Autodesk Inventor part; units mm, degrees
(part 2 of 2)
extrude "Extrusion4" cut sketch "Sketch10" against normal through all contours L3 L2 L1 L0 | L7 L6 L5 L4 | L13 L12 L11 L10 | L17 L16 L15 L14 | L69 L68 L67 L66 | L73 L72 L71 L70 | L77 L76 L75 L74 | L81 L80 L79 L78 | L85 L84 L83 L82 | L89 L88 L87 L86 | L93 L92 L91 L90 | L97 L96 L95 L94 | L101 L100 L99 L98 | L105 L104 L103 L102 | L109 L108 L107 L106 | L113 L112 L111 L110 | L117 L116 L115 L114 | L121 L120 L119 L118 | L125 L124 L123 L122 | L129 L128 L127 L126 | L133 L132 L131 L130 | L137 L136 L135 L134 | L141 L140 L139 L138 | L145 L144 L143 L142 | L197 L196 L195 L194 | L201 L200 L199 L198 | L205 L204 L203 L202 | L209 L208 L207 L206 | L213 L212 L211 L210 | L217 L216 L215 L214 | L221 L220 L219 L218 | L225 L224 L223 L222 | L229 L228 L227 L226 | L233 L232 L231 L230 | L237 L236 L235 L234 | L241 L240 L239 L238 | L245 L244 L243 L242 | L249 L248 L247 L246 | L253 L252 L251 L250 | L257 L256 L255 L254 | L261 L260 L259 L258 | L265 L264 L263 L262 | L269 L268 L267 L266 | L273 L272 L271 L270 | L325 L324 L323 L322 | L329 L328 L327 L326 | L333 L332 L331 L330 | L337 L336 L335 L334 | L341 L340 L339 L338 | L345 L344 L343 L342 | L349 L348 L347 L346 | L353 L352 L351 L350 | L357 L356 L355 L354 | L361 L360 L359 L358 | L365 L364 L363 L362 | L369 L368 L367 L366 | L373 L372 L371 L370 | L377 L376 L375 L374 | L381 L380 L379 L378 | L385 L384 L383 L382 | L389 L388 L387 L386 | L393 L392 L391 L390 | L397 L396 L395 L394 | L401 L400 L399 L398 | L453 L452 L451 L450 | L457 L456 L455 L454 | L461 L460 L459 L458 | L465 L464 L463 L462 | L469 L468 L467 L466 | L473 L472 L471 L470 | L477 L476 L475 L474 | L481 L480 L479 L478 | L485 L484 L483 L482 | L489 L488 L487 L486 | L493 L492 L491 L490 | L497 L496 L495 L494 | L501 L500 L499 L498 | L505 L504 L503 L502 | L509 L508 L507 L506 | L513 L512 L511 L510 | L517 L516 L515 L514 | L521 L520 L519 L518 | L525 L524 L523 L522 | L529 L528 L527 L526 | L533 L532 L531 L530 | L561 L560 L559 L558 | L565 L564 L563 L562 | L585 L584 L583 L582 | L589 L588 L587 L586 | L617 L616 L615 L614 | L621 L620 L619 L618 | L641 L640 L639 L638 | L645 L644 L643 L642 | L649 L648 L647 L646 | L653 L652 L651 L650 | L657 L656 L655 L654 | L661 L660 L659 L658 | L665 L664 L663 L662 | L669 L668 L667 L666 | L673 L672 L671 L670 | L677 L676 L675 L674 | L681 L680 L679 L678 | L685 L684 L683 L682 | L689 L688 L687 L686 | L693 L692 L691 L690 | L697 L696 L695 L694 | L701 L700 L699 L698 | L705 L704 L703 L702 | L709 L708 L707 L706 | L713 L712 L711 L710 | L717 L716 L715 L714 | L721 L720 L719 L718 | L725 L724 L723 L722 | L729 L728 L727 L726 | L733 L732 L731 L730 | L737 L736 L735 L734 | L741 L740 L739 L738 | L745 L744 L743 L742 | L749 L748 L747 L746 | L753 L752 L751 L750 | L757 L756 L755 L754 | L761 L760 L759 L758 | L765 L764 L763 L762 | L769 L768 L767 L766 | L773 L772 L771 L770 | L777 L776 L775 L774 | L781 L780 L779 L778 | L785 L784 L783 L782 | L789 L788 L787 L786 | L793 L792 L791 L790 | L797 L796 L795 L794 | L801 L800 L799 L798 | L805 L804 L803 L802 | L809 L808 L807 L806 | L813 L812 L811 L810 | L817 L816 L815 L814 | L821 L820 L819 L818 | L825 L824 L823 L822 | L829 L828 L827 L826 | L833 L832 L831 L830 | L837 L836 L835 L834 | L841 L840 L839 L838 | L845 L844 L843 L842 | L849 L848 L847 L846 | L853 L852 L851 L850 | L857 L856 L855 L854 | L861 L860 L859 L858 | L865 L864 L863 L862 | L869 L868 L867 L866 | L873 L872 L871 L870 | L877 L876 L875 L874 | L881 L880 L879 L878 | L885 L884 L883 L882 | L889 L888 L887 L886 | L893 L892 L891 L890 | L897 L896 L895 L894 | L901 L900 L899 L898 | L903 L904 L905 L906 | L910 L909 L908 L907 | L914 L913 L912 L911 | L918 L917 L916 L915 | L922 L921 L920 L919 | L926 L925 L924 L923 | L930 L929 L928 L927 | L934 L933 L932 L931 | L938 L937 L936 L935 | L942 L941 L940 L939 | L946 L945 L944 L943
sketch "Sketch15" plane through (0, 4, 0) normal (0, 1, 0) x (1, 0, 0)
  line L0 (-51, 1.5) -> (-22, 1.5)
  line L1 (-22, 1.5) -> (-22, 30.5)
  line L2 (-22, 30.5) -> (-51, 30.5)
  line L3 (-51, 30.5) -> (-51, 1.5)
  line L4 (-39.75, 1.5) -> (-48.25, 1.5) projected
  line L5 (-62, 131.5) -> (-62, -129.5) projected
  line L6 (-51, 31.5) -> (-22, 31.5)
  line L7 (-22, 31.5) -> (-22, 60.5)
  line L8 (-22, 60.5) -> (-51, 60.5)
  line L9 (-51, 60.5) -> (-51, 31.5)
  line L10 (-51, 61.5) -> (-22, 61.5)
  line L11 (-22, 61.5) -> (-22, 90.5)
  line L12 (-22, 90.5) -> (-51, 90.5)
  line L13 (-51, 90.5) -> (-51, 61.5)
  line L14 (-51, 91.5) -> (-22, 91.5)
  line L15 (-22, 91.5) -> (-22, 120.5)
  line L16 (-22, 120.5) -> (-51, 120.5)
  line L17 (-51, 120.5) -> (-51, 91.5)
  line L18 (-39.75, 31.5) -> (-48.25, 31.5) projected
  line L19 (-39.75, 61.5) -> (-48.25, 61.5) projected
  line L20 (-39.75, 91.5) -> (-48.25, 91.5) projected
  point P0 (0, 0)
  dimension "d162" = 29
  dimension "d163" = 0
  dimension "d164" = 11
  dimension "d165" = 29
  dimension "d166" = 29
  dimension "d167" = 29
  dimension "d168" = 29
  dimension "d169" = 0
  dimension "d170" = 0
  dimension "d171" = 0
  dimension "d172" = 11
  constraints: 32 end point, 8 parallel, 5 point on line, 4 horizontal, 4 perpendicular
  measures "d162" distance of L2.end L0.start
  measures "d163" distance between parallel lines of L4 L0
  measures "d164" distance between parallel lines of L5 L3
  measures "d165" distance of L1.end L2.end
  measures "d166" distance of L8.end L6.start
  measures "d167" distance of L12.end L10.start
  measures "d168" distance of L16.end L14.start
  measures "d169" distance between parallel lines of L18 L6
  measures "d170" distance between parallel lines of L19 L10
  measures "d171" distance between parallel lines of L20 L14
  measures "d172" distance between parallel lines of L5 L9
extrude "Extrusion5" cut sketch "Sketch15" against normal through all
sketch "Sketch16" plane through (0, 4, 0) normal (0, 1, 0) x (1, 0, 0)
  line L0 (-51, 0.5) -> (-51, -88.5) projected
  line L1 (-51, 0.5) -> (-22, 0.5)
  line L2 (-22, 0.5) -> (-22, 120.5)
  line L3 (-22, 120.5) -> (-51, 120.5)
  line L4 (-51, 120.5) -> (-51, 0.5)
  point P0 (0, 0)
  constraints: 8 end point, 2 parallel, 1 horizontal, 1 perpendicular
extrude "Extrusion6" cut sketch "Sketch16" against normal through all
sketch "Sketch18" plane through (0, 4, 0) normal (0, 1, 0) x (1, 0, 0)
  line L0 (-38.5, -115.5) -> (-37, -115.5)
  line L1 (-37, -115.5) -> (-37, -107.5)
  line L2 (-37, -107.5) -> (-38.5, -107.5)
  line L3 (-38.5, -107.5) -> (-38.5, -115.5)
  line L4 (-39.75, -118.5) -> (-48.25, -118.5) projected
  line L5 (-39.75, -117) -> (-39.75, -118.5) projected
  line L6 (-23.5, -115.5) -> (-22, -115.5)
  line L7 (-22, -115.5) -> (-22, -107.5)
  line L8 (-22, -107.5) -> (-23.5, -107.5)
  line L9 (-23.5, -107.5) -> (-23.5, -115.5)
  line L10 (-8.5, -115.5) -> (-7, -115.5)
  line L11 (-7, -115.5) -> (-7, -107.5)
  line L12 (-7, -107.5) -> (-8.5, -107.5)
  line L13 (-8.5, -107.5) -> (-8.5, -115.5)
  line L14 (6.5, -115.5) -> (8, -115.5)
  line L15 (8, -115.5) -> (8, -107.5)
  line L16 (8, -107.5) -> (6.5, -107.5)
  line L17 (6.5, -107.5) -> (6.5, -115.5)
  line L18 (21.5, -115.5) -> (23, -115.5)
  line L19 (23, -115.5) -> (23, -107.5)
  line L20 (23, -107.5) -> (21.5, -107.5)
  line L21 (21.5, -107.5) -> (21.5, -115.5)
  line L22 (36.5, -115.5) -> (38, -115.5)
  line L23 (38, -115.5) -> (38, -107.5)
  line L24 (38, -107.5) -> (36.5, -107.5)
  line L25 (36.5, -107.5) -> (36.5, -115.5)
  line L26 (51.5, -115.5) -> (53, -115.5)
  line L27 (53, -115.5) -> (53, -107.5)
  line L28 (53, -107.5) -> (51.5, -107.5)
  line L29 (51.5, -107.5) -> (51.5, -115.5)
  line L30 (-38.5, -100.5) -> (-37, -100.5)
  line L31 (-37, -100.5) -> (-37, -92.5)
  line L32 (-37, -92.5) -> (-38.5, -92.5)
  line L33 (-38.5, -92.5) -> (-38.5, -100.5)
  line L34 (-23.5, -100.5) -> (-22, -100.5)
  line L35 (-22, -100.5) -> (-22, -92.5)
  line L36 (-22, -92.5) -> (-23.5, -92.5)
  line L37 (-23.5, -92.5) -> (-23.5, -100.5)
  line L38 (-8.5, -100.5) -> (-7, -100.5)
  line L39 (-7, -100.5) -> (-7, -92.5)
  line L40 (-7, -92.5) -> (-8.5, -92.5)
  line L41 (-8.5, -92.5) -> (-8.5, -100.5)
  line L42 (6.5, -100.5) -> (8, -100.5)
  line L43 (8, -100.5) -> (8, -92.5)
  line L44 (8, -92.5) -> (6.5, -92.5)
  line L45 (6.5, -92.5) -> (6.5, -100.5)
  line L46 (21.5, -100.5) -> (23, -100.5)
  line L47 (23, -100.5) -> (23, -92.5)
  line L48 (23, -92.5) -> (21.5, -92.5)
  line L49 (21.5, -92.5) -> (21.5, -100.5)
  line L50 (36.5, -100.5) -> (38, -100.5)
  line L51 (38, -100.5) -> (38, -92.5)
  line L52 (38, -92.5) -> (36.5, -92.5)
  line L53 (36.5, -92.5) -> (36.5, -100.5)
  line L54 (51.5, -100.5) -> (53, -100.5)
  line L55 (53, -100.5) -> (53, -92.5)
  line L56 (53, -92.5) -> (51.5, -92.5)
  line L57 (51.5, -92.5) -> (51.5, -100.5)
  line L58 (-38.5, -85.5) -> (-37, -85.5)
  line L59 (-37, -85.5) -> (-37, -77.5)
  line L60 (-37, -77.5) -> (-38.5, -77.5)
  line L61 (-38.5, -77.5) -> (-38.5, -85.5)
  line L62 (-23.5, -85.5) -> (-22, -85.5)
  line L63 (-22, -85.5) -> (-22, -77.5)
  line L64 (-22, -77.5) -> (-23.5, -77.5)
  line L65 (-23.5, -77.5) -> (-23.5, -85.5)
  line L66 (-8.5, -85.5) -> (-7, -85.5)
  line L67 (-7, -85.5) -> (-7, -77.5)
  line L68 (-7, -77.5) -> (-8.5, -77.5)
  line L69 (-8.5, -77.5) -> (-8.5, -85.5)
  line L70 (6.5, -85.5) -> (8, -85.5)
  line L71 (8, -85.5) -> (8, -77.5)
  line L72 (8, -77.5) -> (6.5, -77.5)
  line L73 (6.5, -77.5) -> (6.5, -85.5)
  line L74 (21.5, -85.5) -> (23, -85.5)
  line L75 (23, -85.5) -> (23, -77.5)
  line L76 (23, -77.5) -> (21.5, -77.5)
  line L77 (21.5, -77.5) -> (21.5, -85.5)
  line L78 (36.5, -85.5) -> (38, -85.5)
  line L79 (38, -85.5) -> (38, -77.5)
  line L80 (38, -77.5) -> (36.5, -77.5)
  line L81 (36.5, -77.5) -> (36.5, -85.5)
  line L82 (51.5, -85.5) -> (53, -85.5)
  line L83 (53, -85.5) -> (53, -77.5)
  line L84 (53, -77.5) -> (51.5, -77.5)
  line L85 (51.5, -77.5) -> (51.5, -85.5)
  line L86 (-38.5, -70.5) -> (-37, -70.5)
  line L87 (-37, -70.5) -> (-37, -62.5)
  line L88 (-37, -62.5) -> (-38.5, -62.5)
  line L89 (-38.5, -62.5) -> (-38.5, -70.5)
  line L90 (-23.5, -70.5) -> (-22, -70.5)
  line L91 (-22, -70.5) -> (-22, -62.5)
  line L92 (-22, -62.5) -> (-23.5, -62.5)
  line L93 (-23.5, -62.5) -> (-23.5, -70.5)
  line L94 (-8.5, -70.5) -> (-7, -70.5)
  line L95 (-7, -70.5) -> (-7, -62.5)
  line L96 (-7, -62.5) -> (-8.5, -62.5)
  line L97 (-8.5, -62.5) -> (-8.5, -70.5)
  line L98 (6.5, -70.5) -> (8, -70.5)
  line L99 (8, -70.5) -> (8, -62.5)
  line L100 (8, -62.5) -> (6.5, -62.5)
  line L101 (6.5, -62.5) -> (6.5, -70.5)
  line L102 (21.5, -70.5) -> (23, -70.5)
  line L103 (23, -70.5) -> (23, -62.5)
  line L104 (23, -62.5) -> (21.5, -62.5)
  line L105 (21.5, -62.5) -> (21.5, -70.5)
  line L106 (36.5, -70.5) -> (38, -70.5)
  line L107 (38, -70.5) -> (38, -62.5)
  line L108 (38, -62.5) -> (36.5, -62.5)
  line L109 (36.5, -62.5) -> (36.5, -70.5)
  line L110 (51.5, -70.5) -> (53, -70.5)
  line L111 (53, -70.5) -> (53, -62.5)
  line L112 (53, -62.5) -> (51.5, -62.5)
  line L113 (51.5, -62.5) -> (51.5, -70.5)
  line L114 (-38.5, -55.5) -> (-37, -55.5)
  line L115 (-37, -55.5) -> (-37, -47.5)
  line L116 (-37, -47.5) -> (-38.5, -47.5)
  line L117 (-38.5, -47.5) -> (-38.5, -55.5)
  line L118 (-23.5, -55.5) -> (-22, -55.5)
  line L119 (-22, -55.5) -> (-22, -47.5)
  line L120 (-22, -47.5) -> (-23.5, -47.5)
  line L121 (-23.5, -47.5) -> (-23.5, -55.5)
  line L122 (-8.5, -55.5) -> (-7, -55.5)
  line L123 (-7, -55.5) -> (-7, -47.5)
  line L124 (-7, -47.5) -> (-8.5, -47.5)
  line L125 (-8.5, -47.5) -> (-8.5, -55.5)
  line L126 (6.5, -55.5) -> (8, -55.5)
  line L127 (8, -55.5) -> (8, -47.5)
  line L128 (8, -47.5) -> (6.5, -47.5)
  line L129 (6.5, -47.5) -> (6.5, -55.5)
  line L130 (21.5, -55.5) -> (23, -55.5)
  line L131 (23, -55.5) -> (23, -47.5)
  line L132 (23, -47.5) -> (21.5, -47.5)
  line L133 (21.5, -47.5) -> (21.5, -55.5)
  line L134 (36.5, -55.5) -> (38, -55.5)
  line L135 (38, -55.5) -> (38, -47.5)
  line L136 (38, -47.5) -> (36.5, -47.5)
  line L137 (36.5, -47.5) -> (36.5, -55.5)
  line L138 (51.5, -55.5) -> (53, -55.5)
  line L139 (53, -55.5) -> (53, -47.5)
  line L140 (53, -47.5) -> (51.5, -47.5)
  line L141 (51.5, -47.5) -> (51.5, -55.5)
  line L142 (-38.5, -40.5) -> (-37, -40.5)
  line L143 (-37, -40.5) -> (-37, -32.5)
  line L144 (-37, -32.5) -> (-38.5, -32.5)
  line L145 (-38.5, -32.5) -> (-38.5, -40.5)
  line L146 (-23.5, -40.5) -> (-22, -40.5)
  line L147 (-22, -40.5) -> (-22, -32.5)
  line L148 (-22, -32.5) -> (-23.5, -32.5)
  line L149 (-23.5, -32.5) -> (-23.5, -40.5)
  line L150 (-8.5, -40.5) -> (-7, -40.5)
  line L151 (-7, -40.5) -> (-7, -32.5)
  line L152 (-7, -32.5) -> (-8.5, -32.5)
  line L153 (-8.5, -32.5) -> (-8.5, -40.5)
  line L154 (6.5, -40.5) -> (8, -40.5)
  line L155 (8, -40.5) -> (8, -32.5)
  line L156 (8, -32.5) -> (6.5, -32.5)
  line L157 (6.5, -32.5) -> (6.5, -40.5)
  line L158 (21.5, -40.5) -> (23, -40.5)
  line L159 (23, -40.5) -> (23, -32.5)
  line L160 (23, -32.5) -> (21.5, -32.5)
  line L161 (21.5, -32.5) -> (21.5, -40.5)
  line L162 (36.5, -40.5) -> (38, -40.5)
  line L163 (38, -40.5) -> (38, -32.5)
  line L164 (38, -32.5) -> (36.5, -32.5)
  line L165 (36.5, -32.5) -> (36.5, -40.5)
  line L166 (51.5, -40.5) -> (53, -40.5)
  line L167 (53, -40.5) -> (53, -32.5)
  line L168 (53, -32.5) -> (51.5, -32.5)
  line L169 (51.5, -32.5) -> (51.5, -40.5)
  line L170 (-38.5, -25.5) -> (-37, -25.5)
  line L171 (-37, -25.5) -> (-37, -17.5)
  line L172 (-37, -17.5) -> (-38.5, -17.5)
  line L173 (-38.5, -17.5) -> (-38.5, -25.5)
  line L174 (-23.5, -25.5) -> (-22, -25.5)
  line L175 (-22, -25.5) -> (-22, -17.5)
  line L176 (-22, -17.5) -> (-23.5, -17.5)
  line L177 (-23.5, -17.5) -> (-23.5, -25.5)
  line L178 (-8.5, -25.5) -> (-7, -25.5)
  line L179 (-7, -25.5) -> (-7, -17.5)
  line L180 (-7, -17.5) -> (-8.5, -17.5)
  line L181 (-8.5, -17.5) -> (-8.5, -25.5)
  line L182 (6.5, -25.5) -> (8, -25.5)
  line L183 (8, -25.5) -> (8, -17.5)
  line L184 (8, -17.5) -> (6.5, -17.5)
  line L185 (6.5, -17.5) -> (6.5, -25.5)
  line L186 (21.5, -25.5) -> (23, -25.5)
  line L187 (23, -25.5) -> (23, -17.5)
  line L188 (23, -17.5) -> (21.5, -17.5)
  line L189 (21.5, -17.5) -> (21.5, -25.5)
  line L190 (36.5, -25.5) -> (38, -25.5)
  line L191 (38, -25.5) -> (38, -17.5)
  line L192 (38, -17.5) -> (36.5, -17.5)
  line L193 (36.5, -17.5) -> (36.5, -25.5)
  line L194 (51.5, -25.5) -> (53, -25.5)
  line L195 (53, -25.5) -> (53, -17.5)
  line L196 (53, -17.5) -> (51.5, -17.5)
  line L197 (51.5, -17.5) -> (51.5, -25.5)
  line L198 (-38.5, -10.5) -> (-37, -10.5)
  line L199 (-37, -10.5) -> (-37, -2.5)
  line L200 (-37, -2.5) -> (-38.5, -2.5)
  line L201 (-38.5, -2.5) -> (-38.5, -10.5)
  line L202 (-23.5, -10.5) -> (-22, -10.5)
  line L203 (-22, -10.5) -> (-22, -2.5)
  line L204 (-22, -2.5) -> (-23.5, -2.5)
  line L205 (-23.5, -2.5) -> (-23.5, -10.5)
  line L206 (-8.5, -10.5) -> (-7, -10.5)
  line L207 (-7, -10.5) -> (-7, -2.5)
  line L208 (-7, -2.5) -> (-8.5, -2.5)
  line L209 (-8.5, -2.5) -> (-8.5, -10.5)
  line L210 (6.5, -10.5) -> (8, -10.5)
  line L211 (8, -10.5) -> (8, -2.5)
  line L212 (8, -2.5) -> (6.5, -2.5)
  line L213 (6.5, -2.5) -> (6.5, -10.5)
  line L214 (21.5, -10.5) -> (23, -10.5)
  line L215 (23, -10.5) -> (23, -2.5)
  line L216 (23, -2.5) -> (21.5, -2.5)
  line L217 (21.5, -2.5) -> (21.5, -10.5)
  line L218 (36.5, -10.5) -> (38, -10.5)
  line L219 (38, -10.5) -> (38, -2.5)
  line L220 (38, -2.5) -> (36.5, -2.5)
  line L221 (36.5, -2.5) -> (36.5, -10.5)
  line L222 (51.5, -10.5) -> (53, -10.5)
  line L223 (53, -10.5) -> (53, -2.5)
  line L224 (53, -2.5) -> (51.5, -2.5)
  line L225 (51.5, -2.5) -> (51.5, -10.5)
  line L226 (-38.5, 4.5) -> (-37, 4.5)
  line L227 (-37, 4.5) -> (-37, 12.5)
  line L228 (-37, 12.5) -> (-38.5, 12.5)
  line L229 (-38.5, 12.5) -> (-38.5, 4.5)
  line L230 (-23.5, 4.5) -> (-22, 4.5)
  line L231 (-22, 4.5) -> (-22, 12.5)
  line L232 (-22, 12.5) -> (-23.5, 12.5)
  line L233 (-23.5, 12.5) -> (-23.5, 4.5)
  line L234 (-8.5, 4.5) -> (-7, 4.5)
  line L235 (-7, 4.5) -> (-7, 12.5)
  line L236 (-7, 12.5) -> (-8.5, 12.5)
  line L237 (-8.5, 12.5) -> (-8.5, 4.5)
  line L238 (6.5, 4.5) -> (8, 4.5)
  line L239 (8, 4.5) -> (8, 12.5)
  line L240 (8, 12.5) -> (6.5, 12.5)
  line L241 (6.5, 12.5) -> (6.5, 4.5)
  line L242 (21.5, 4.5) -> (23, 4.5)
  line L243 (23, 4.5) -> (23, 12.5)
  line L244 (23, 12.5) -> (21.5, 12.5)
  line L245 (21.5, 12.5) -> (21.5, 4.5)
  line L246 (36.5, 4.5) -> (38, 4.5)
  line L247 (38, 4.5) -> (38, 12.5)
  line L248 (38, 12.5) -> (36.5, 12.5)
  line L249 (36.5, 12.5) -> (36.5, 4.5)
  line L250 (51.5, 4.5) -> (53, 4.5)
  line L251 (53, 4.5) -> (53, 12.5)
  line L252 (53, 12.5) -> (51.5, 12.5)
  line L253 (51.5, 12.5) -> (51.5, 4.5)
  line L254 (-38.5, 19.5) -> (-37, 19.5)
  line L255 (-37, 19.5) -> (-37, 27.5)
  line L256 (-37, 27.5) -> (-38.5, 27.5)
  line L257 (-38.5, 27.5) -> (-38.5, 19.5)
  line L258 (-23.5, 19.5) -> (-22, 19.5)
  line L259 (-22, 19.5) -> (-22, 27.5)
  line L260 (-22, 27.5) -> (-23.5, 27.5)
  line L261 (-23.5, 27.5) -> (-23.5, 19.5)
  line L262 (-8.5, 19.5) -> (-7, 19.5)
  line L263 (-7, 19.5) -> (-7, 27.5)
  line L264 (-7, 27.5) -> (-8.5, 27.5)
  line L265 (-8.5, 27.5) -> (-8.5, 19.5)
  line L266 (6.5, 19.5) -> (8, 19.5)
  line L267 (8, 19.5) -> (8, 27.5)
  line L268 (8, 27.5) -> (6.5, 27.5)
  line L269 (6.5, 27.5) -> (6.5, 19.5)
  line L270 (21.5, 19.5) -> (23, 19.5)
  line L271 (23, 19.5) -> (23, 27.5)
  line L272 (23, 27.5) -> (21.5, 27.5)
  line L273 (21.5, 27.5) -> (21.5, 19.5)
  line L274 (36.5, 19.5) -> (38, 19.5)
  line L275 (38, 19.5) -> (38, 27.5)
  line L276 (38, 27.5) -> (36.5, 27.5)
  line L277 (36.5, 27.5) -> (36.5, 19.5)
  line L278 (51.5, 19.5) -> (53, 19.5)
  line L279 (53, 19.5) -> (53, 27.5)
  line L280 (53, 27.5) -> (51.5, 27.5)
  line L281 (51.5, 27.5) -> (51.5, 19.5)
  line L282 (-38.5, 34.5) -> (-37, 34.5)
  line L283 (-37, 34.5) -> (-37, 42.5)
  line L284 (-37, 42.5) -> (-38.5, 42.5)
  line L285 (-38.5, 42.5) -> (-38.5, 34.5)
  line L286 (-23.5, 34.5) -> (-22, 34.5)
  line L287 (-22, 34.5) -> (-22, 42.5)
  line L288 (-22, 42.5) -> (-23.5, 42.5)
  line L289 (-23.5, 42.5) -> (-23.5, 34.5)
  line L290 (-8.5, 34.5) -> (-7, 34.5)
  line L291 (-7, 34.5) -> (-7, 42.5)
  line L292 (-7, 42.5) -> (-8.5, 42.5)
  line L293 (-8.5, 42.5) -> (-8.5, 34.5)
  line L294 (6.5, 34.5) -> (8, 34.5)
  line L295 (8, 34.5) -> (8, 42.5)
  line L296 (8, 42.5) -> (6.5, 42.5)
  line L297 (6.5, 42.5) -> (6.5, 34.5)
  line L298 (21.5, 34.5) -> (23, 34.5)
  line L299 (23, 34.5) -> (23, 42.5)
  line L300 (23, 42.5) -> (21.5, 42.5)
  line L301 (21.5, 42.5) -> (21.5, 34.5)
  line L302 (36.5, 34.5) -> (38, 34.5)
  line L303 (38, 34.5) -> (38, 42.5)
  line L304 (38, 42.5) -> (36.5, 42.5)
  line L305 (36.5, 42.5) -> (36.5, 34.5)
  line L306 (51.5, 34.5) -> (53, 34.5)
  line L307 (53, 34.5) -> (53, 42.5)
  line L308 (53, 42.5) -> (51.5, 42.5)
  line L309 (51.5, 42.5) -> (51.5, 34.5)
  line L310 (-38.5, 49.5) -> (-37, 49.5)
  line L311 (-37, 49.5) -> (-37, 57.5)
  line L312 (-37, 57.5) -> (-38.5, 57.5)
  line L313 (-38.5, 57.5) -> (-38.5, 49.5)
  line L314 (-23.5, 49.5) -> (-22, 49.5)
  line L315 (-22, 49.5) -> (-22, 57.5)
  line L316 (-22, 57.5) -> (-23.5, 57.5)
  line L317 (-23.5, 57.5) -> (-23.5, 49.5)
  line L318 (-8.5, 49.5) -> (-7, 49.5)
  line L319 (-7, 49.5) -> (-7, 57.5)
  line L320 (-7, 57.5) -> (-8.5, 57.5)
  line L321 (-8.5, 57.5) -> (-8.5, 49.5)
  line L322 (6.5, 49.5) -> (8, 49.5)
  line L323 (8, 49.5) -> (8, 57.5)
  line L324 (8, 57.5) -> (6.5, 57.5)
  line L325 (6.5, 57.5) -> (6.5, 49.5)
  line L326 (21.5, 49.5) -> (23, 49.5)
  line L327 (23, 49.5) -> (23, 57.5)
  line L328 (23, 57.5) -> (21.5, 57.5)
  line L329 (21.5, 57.5) -> (21.5, 49.5)
  line L330 (36.5, 49.5) -> (38, 49.5)
  line L331 (38, 49.5) -> (38, 57.5)
  line L332 (38, 57.5) -> (36.5, 57.5)
  line L333 (36.5, 57.5) -> (36.5, 49.5)
  line L334 (51.5, 49.5) -> (53, 49.5)
  line L335 (53, 49.5) -> (53, 57.5)
  line L336 (53, 57.5) -> (51.5, 57.5)
  line L337 (51.5, 57.5) -> (51.5, 49.5)
  line L338 (-38.5, 64.5) -> (-37, 64.5)
  line L339 (-37, 64.5) -> (-37, 72.5)
  line L340 (-37, 72.5) -> (-38.5, 72.5)
  line L341 (-38.5, 72.5) -> (-38.5, 64.5)
  line L342 (-23.5, 64.5) -> (-22, 64.5)
  line L343 (-22, 64.5) -> (-22, 72.5)
  line L344 (-22, 72.5) -> (-23.5, 72.5)
  line L345 (-23.5, 72.5) -> (-23.5, 64.5)
  line L346 (-8.5, 64.5) -> (-7, 64.5)
  line L347 (-7, 64.5) -> (-7, 72.5)
  line L348 (-7, 72.5) -> (-8.5, 72.5)
  line L349 (-8.5, 72.5) -> (-8.5, 64.5)
  line L350 (6.5, 64.5) -> (8, 64.5)
  line L351 (8, 64.5) -> (8, 72.5)
  line L352 (8, 72.5) -> (6.5, 72.5)
  line L353 (6.5, 72.5) -> (6.5, 64.5)
  line L354 (21.5, 64.5) -> (23, 64.5)
  line L355 (23, 64.5) -> (23, 72.5)
  line L356 (23, 72.5) -> (21.5, 72.5)
  line L357 (21.5, 72.5) -> (21.5, 64.5)
  line L358 (36.5, 64.5) -> (38, 64.5)
  line L359 (38, 64.5) -> (38, 72.5)
  line L360 (38, 72.5) -> (36.5, 72.5)
  line L361 (36.5, 72.5) -> (36.5, 64.5)
  line L362 (51.5, 64.5) -> (53, 64.5)
  line L363 (53, 64.5) -> (53, 72.5)
  line L364 (53, 72.5) -> (51.5, 72.5)
  line L365 (51.5, 72.5) -> (51.5, 64.5)
  line L366 (-38.5, 79.5) -> (-37, 79.5)
  line L367 (-37, 79.5) -> (-37, 87.5)
  line L368 (-37, 87.5) -> (-38.5, 87.5)
  line L369 (-38.5, 87.5) -> (-38.5, 79.5)
  line L370 (-23.5, 79.5) -> (-22, 79.5)
  line L371 (-22, 79.5) -> (-22, 87.5)
  line L372 (-22, 87.5) -> (-23.5, 87.5)
  line L373 (-23.5, 87.5) -> (-23.5, 79.5)
  line L374 (-8.5, 79.5) -> (-7, 79.5)
  line L375 (-7, 79.5) -> (-7, 87.5)
  line L376 (-7, 87.5) -> (-8.5, 87.5)
  line L377 (-8.5, 87.5) -> (-8.5, 79.5)
  line L378 (6.5, 79.5) -> (8, 79.5)
  line L379 (8, 79.5) -> (8, 87.5)
  line L380 (8, 87.5) -> (6.5, 87.5)
  line L381 (6.5, 87.5) -> (6.5, 79.5)
  line L382 (21.5, 79.5) -> (23, 79.5)
  line L383 (23, 79.5) -> (23, 87.5)
  line L384 (23, 87.5) -> (21.5, 87.5)
  line L385 (21.5, 87.5) -> (21.5, 79.5)
  line L386 (36.5, 79.5) -> (38, 79.5)
  line L387 (38, 79.5) -> (38, 87.5)
  line L388 (38, 87.5) -> (36.5, 87.5)
  line L389 (36.5, 87.5) -> (36.5, 79.5)
  line L390 (51.5, 79.5) -> (53, 79.5)
  line L391 (53, 79.5) -> (53, 87.5)
  line L392 (53, 87.5) -> (51.5, 87.5)
  line L393 (51.5, 87.5) -> (51.5, 79.5)
  line L394 (-38.5, 94.5) -> (-37, 94.5)
  line L395 (-37, 94.5) -> (-37, 102.5)
  line L396 (-37, 102.5) -> (-38.5, 102.5)
  line L397 (-38.5, 102.5) -> (-38.5, 94.5)
  line L398 (-23.5, 94.5) -> (-22, 94.5)
  line L399 (-22, 94.5) -> (-22, 102.5)
  line L400 (-22, 102.5) -> (-23.5, 102.5)
  line L401 (-23.5, 102.5) -> (-23.5, 94.5)
  line L402 (-8.5, 94.5) -> (-7, 94.5)
  line L403 (-7, 94.5) -> (-7, 102.5)
  line L404 (-7, 102.5) -> (-8.5, 102.5)
  line L405 (-8.5, 102.5) -> (-8.5, 94.5)
  line L406 (6.5, 94.5) -> (8, 94.5)
  line L407 (8, 94.5) -> (8, 102.5)
  line L408 (8, 102.5) -> (6.5, 102.5)
  line L409 (6.5, 102.5) -> (6.5, 94.5)
  line L410 (21.5, 94.5) -> (23, 94.5)
  line L411 (23, 94.5) -> (23, 102.5)
  line L412 (23, 102.5) -> (21.5, 102.5)
  line L413 (21.5, 102.5) -> (21.5, 94.5)
  line L414 (36.5, 94.5) -> (38, 94.5)
  line L415 (38, 94.5) -> (38, 102.5)
  line L416 (38, 102.5) -> (36.5, 102.5)
  line L417 (36.5, 102.5) -> (36.5, 94.5)
  line L418 (51.5, 94.5) -> (53, 94.5)
  line L419 (53, 94.5) -> (53, 102.5)
  line L420 (53, 102.5) -> (51.5, 102.5)
  line L421 (51.5, 102.5) -> (51.5, 94.5)
  line L422 (-38.5, 109.5) -> (-37, 109.5)
  line L423 (-37, 109.5) -> (-37, 117.5)
  line L424 (-37, 117.5) -> (-38.5, 117.5)
  line L425 (-38.5, 117.5) -> (-38.5, 109.5)
  line L426 (-23.5, 109.5) -> (-22, 109.5)
  line L427 (-22, 109.5) -> (-22, 117.5)
  line L428 (-22, 117.5) -> (-23.5, 117.5)
  line L429 (-23.5, 117.5) -> (-23.5, 109.5)
  line L430 (-8.5, 109.5) -> (-7, 109.5)
  line L431 (-7, 109.5) -> (-7, 117.5)
  line L432 (-7, 117.5) -> (-8.5, 117.5)
  line L433 (-8.5, 117.5) -> (-8.5, 109.5)
  line L434 (6.5, 109.5) -> (8, 109.5)
  line L435 (8, 109.5) -> (8, 117.5)
  line L436 (8, 117.5) -> (6.5, 117.5)
  line L437 (6.5, 117.5) -> (6.5, 109.5)
  line L438 (21.5, 109.5) -> (23, 109.5)
  line L439 (23, 109.5) -> (23, 117.5)
  line L440 (23, 117.5) -> (21.5, 117.5)
  line L441 (21.5, 117.5) -> (21.5, 109.5)
  line L442 (36.5, 109.5) -> (38, 109.5)
  line L443 (38, 109.5) -> (38, 117.5)
  line L444 (38, 117.5) -> (36.5, 117.5)
  line L445 (36.5, 117.5) -> (36.5, 109.5)
  line L446 (51.5, 109.5) -> (53, 109.5)
  line L447 (53, 109.5) -> (53, 117.5)
  line L448 (53, 117.5) -> (51.5, 117.5)
  line L449 (51.5, 117.5) -> (51.5, 109.5)
  line L450 (21.5, -81.75) -> (23, -81.75)
  line L451 (23, -81.75) -> (23, -73.75)
  line L452 (23, -73.75) -> (21.5, -73.75)
  line L453 (21.5, -73.75) -> (21.5, -81.75)
  line L454 (20.25, -88.5) -> (11.75, -88.5) projected
  line L455 (21.5, -63) -> (23, -63)
  line L456 (23, -63) -> (23, -55)
  line L457 (23, -55) -> (21.5, -55)
  line L458 (21.5, -55) -> (21.5, -63)
  line L459 (20.25, -66) -> (11.75, -66) projected
  line L460 (21.5, -36.25) -> (23, -36.25)
  line L461 (23, -36.25) -> (23, -44.25)
  line L462 (23, -44.25) -> (21.5, -44.25)
  line L463 (21.5, -44.25) -> (21.5, -36.25)
  line L464 (20.25, -51) -> (11.75, -51) projected
  line L465 (21.5, -21.75) -> (23, -21.75)
  line L466 (23, -21.75) -> (23, -13.75)
  line L467 (23, -13.75) -> (21.5, -13.75)
  line L468 (21.5, -13.75) -> (21.5, -21.75)
  line L469 (11.75, -7) -> (20.25, -7) projected
  line L470 (21.5, 8.75) -> (23, 8.75)
  line L471 (23, 8.75) -> (23, 0.75)
  line L472 (23, 0.75) -> (21.5, 0.75)
  line L473 (21.5, 0.75) -> (21.5, 8.75)
  line L474 (20.25, -6) -> (11.75, -6) projected
  line L475 (21.5, 23.25) -> (23, 23.25)
  line L476 (23, 23.25) -> (23, 31.25)
  line L477 (23, 31.25) -> (21.5, 31.25)
  line L478 (21.5, 31.25) -> (21.5, 23.25)
  line L479 (11.75, 38) -> (20.25, 38) projected
  line L480 (21.5, 42) -> (23, 42)
  line L481 (23, 42) -> (23, 50)
  line L482 (23, 50) -> (21.5, 50)
  line L483 (21.5, 50) -> (21.5, 42)
  line L484 (20.25, 39) -> (11.75, 39) projected
  line L485 (21.5, 68.75) -> (23, 68.75)
  line L486 (23, 68.75) -> (23, 60.75)
  line L487 (23, 60.75) -> (21.5, 60.75)
  line L488 (21.5, 60.75) -> (21.5, 68.75)
  line L489 (20.25, 54) -> (11.75, 54) projected
  line L490 (21.5, 83.25) -> (23, 83.25)
  line L491 (23, 83.25) -> (23, 91.25)
  line L492 (23, 91.25) -> (21.5, 91.25)
  line L493 (21.5, 91.25) -> (21.5, 83.25)
  line L494 (20.25, 76.5) -> (11.75, 76.5) projected
  line L495 (21.5, 105.75) -> (23, 105.75)
  line L496 (23, 105.75) -> (23, 113.75)
  line L497 (23, 113.75) -> (21.5, 113.75)
  line L498 (21.5, 113.75) -> (21.5, 105.75)
  line L499 (20.25, 99) -> (11.75, 99) projected
  point P0 (0, 0)
  dimension "d177" = 8
  dimension "d178" = 1.5
  dimension "d179" = 3
  dimension "d180" = 1.25
  dimension "d187" = 15
  dimension "d190" = 15
  dimension "d193" = 8
  dimension "d194" = 1.5
  dimension "d195" = 6.75
  dimension "d200" = 8
  dimension "d201" = 3
  dimension "d202" = 1.5
  dimension "d203" = 8
  dimension "d204" = 6.75
  dimension "d205" = 8
  dimension "d206" = 6.75
  dimension "d207" = 1.5
  dimension "d208" = 8
  dimension "d209" = 6.75
  dimension "d210" = 8
  dimension "d211" = 6.75
  dimension "d212" = 8
  dimension "d213" = 3
  dimension "d214" = 8
  dimension "d215" = 6.75
  dimension "d216" = 8
  dimension "d217" = 6.75
  dimension "d218" = 1.5
  dimension "d219" = 8
  dimension "d220" = 6.75
  constraints: 976 end point, 22 parallel, 15 point on line, 12 horizontal, 11 perpendicular, 1 vertical, 888 other
  measures "d177" distance of L2.end L0.start
  measures "d178" distance of L1.end L2.end
  measures "d179" distance between parallel lines of L4 L0
  measures "d180" distance between parallel lines of L5 L3
  measures "d187" distance of L0.start L6.start
  measures "d190" distance of L0.start L30.start
  measures "d193" distance of L450.end L451.end
  measures "d194" distance of L451.end L452.end
  measures "d195" distance between parallel lines of L454 L450
  measures "d200" distance of L455.end L456.end
  measures "d201" distance between parallel lines of L459 L455
  measures "d202" distance of L461.end L462.end
  measures "d203" distance of L460.end L461.end
  measures "d204" distance between parallel lines of L464 L462
  measures "d205" distance of L465.end L466.end
  measures "d206" distance between parallel lines of L469 L467
  measures "d207" distance of L465.start L465.end
  measures "d208" distance of L470.end L471.end
  measures "d209" distance between parallel lines of L474 L472
  measures "d210" distance of L477.end L475.start
  measures "d211" distance between parallel lines of L479 L477
  measures "d212" distance of L482.end L480.start
  measures "d213" distance between parallel lines of L484 L480
  measures "d214" distance of L485.end L486.end
  measures "d215" distance between parallel lines of L489 L487
  measures "d216" distance of L490.end L491.end
  measures "d217" distance between parallel lines of L494 L490
  measures "d218" distance of L491.end L492.end
  measures "d219" distance of L495.end L496.end
  measures "d220" distance between parallel lines of L499 L495
extrude "Extrusion7" cut sketch "Sketch18" against normal blind 8 contours L3 L2 L1 L0 | L9 L8 L7 L6 | L13 L12 L11 L10 | L17 L16 L15 L14 | L21 L20 L19 L18 | L25 L24 L23 L22 | L29 L28 L27 L26 | L33 L32 L31 L30 | L37 L36 L35 L34 | L41 L40 L39 L38 | L45 L44 L43 L42 | L49 L48 L47 L46 | L53 L52 L51 L50 | L57 L56 L55 L54 | L77 L76 L75 L450 | L453 L452 L451 L76 | L81 L80 L79 L78 | L85 L84 L83 L82 | L105 L104 L103 L455 | L458 L130 L456 L104 | L133 L457 L131 L130 | L109 L108 L107 L106 | L113 L112 L111 L110 | L137 L136 L135 L134 | L141 L140 L139 L138 | L161 L460 L159 L158 | L158 L461 L462 L463 | L165 L164 L163 L162 | L169 L168 L167 L166 | L189 L188 L187 L465 | L468 L467 L466 L188 | L193 L192 L191 L190 | L197 L196 L195 L194 | L221 L220 L219 L218 | L225 L224 L223 L222 | L237 L236 L235 L234 | L241 L240 L239 L238 | L245 L470 L243 L242 | L242 L471 L472 L473 | L249 L248 L247 L246 | L253 L252 L251 L250 | L265 L264 L263 L262 | L269 L268 L267 L266 | L273 L272 L271 L475 | L478 L477 L476 L272 | L277 L276 L275 L274 | L281 L280 L279 L278 | L293 L292 L291 L290 | L297 L296 L295 L294 | L301 L300 L299 L480 | L483 L326 L481 L300 | L329 L482 L327 L326 | L305 L304 L303 L302 | L309 L308 L307 L306 | L321 L320 L319 L318 | L325 L324 L323 L322 | L333 L332 L331 L330 | L337 L336 L335 L334 | L349 L348 L347 L346 | L353 L352 L351 L350 | L357 L485 L355 L354 | L354 L486 L487 L488 | L361 L360 L359 L358 | L365 L364 L363 L362 | L377 L376 L375 L374 | L381 L380 L379 L378 | L385 L384 L383 L490 | L493 L492 L491 L384 | L389 L388 L387 L386 | L393 L392 L391 L390 | L405 L404 L403 L402 | L409 L408 L407 L406 | L417 L416 L415 L414 | L421 L420 L419 L418 | L433 L432 L431 L430 | L437 L436 L435 L434 | L441 L497 L439 L438 | L438 L496 L495 L498 | L445 L444 L443 L442 | L449 L448 L447 L446
body "Solid1"
